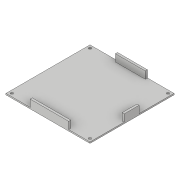
# Autodesk Inventor part: Board
Saved by Autodesk Inventor 2017 (Build 210142000, 142)
## iProperties
Created: 2019-06-10
Part Number: Board
Material: Generic
Document SubType Name: Modeling
Designer: markg
Density: 1 g/cm^3
Appearance: Default
Author: markg
Autodesk Inventor part; units mm, degrees
ref_plane "YZ Plane" through (0, 0, 0) normal (1, 0, 0) x (0, 1, 0)
ref_plane "XZ Plane" through (0, 0, 0) normal (0, 1, 0) x (-1, 0, 0)
ref_plane "XY Plane" through (0, 0, 0) normal (0, 0, 1) x (1, 0, 0)
sketch "Sketch1" plane through (0, 0, 0) normal (0, 1, 0) x (-1, 0, 0)
  line L0 (-50, 50) -> (50, 50)
  line L1 (50, 50) -> (50, -50)
  line L2 (50, -50) -> (-50, -50)
  line L3 (-50, -50) -> (-50, 50)
  line L4 (-50, 50) -> (50, -50) construction
  line L5 (50, 50) -> (-50, -50) construction
  circle A0 centre (46.444, 46.444) radius 1.5875
  circle A1 centre (46.444, -46.444) radius 1.5875
  circle A2 centre (-46.444, -46.444) radius 1.5875
  circle A3 centre (-46.444, 46.444) radius 1.5875
  point P0 (0, 0)
  dimension "d0" = 100
  dimension "d1" = 100
  dimension "d2" = 3.175
  dimension "d3" = 3.175
  dimension "d4" = 3.175
  dimension "d5" = 3.175
  dimension "d6" = 3.556
  dimension "d7" = 3.556
  dimension "d8" = 3.556
  dimension "d9" = 3.556
  constraints: 12 end point, 4 centre point, 4 point on line, 2 midpoint, 2 parallel, 1 horizontal, 1 perpendicular
  measures "d0" distance of L0.end L1.end
  measures "d1" distance of L1.end L2.end
  measures "d2" diameter of A0
  measures "d3" diameter of A1
  measures "d4" diameter of A2
  measures "d5" diameter of A3
  measures "d6" distance from line of L1 A0.centre
  measures "d7" distance from line of L1 A1.centre
  measures "d8" distance from line of L3 A2.centre
  measures "d9" distance from line of L3 A3.centre
extrude "Extrusion1" add sketch "Sketch1" along normal blind 1.5875
sketch "Sketch2" plane through (0, 1.5875, 0) normal (0, 1, 0) x (1, 0, 0)
  line L0 (-21.12, -50) -> (24.6, -50)
  line L1 (24.6, -50) -> (24.6, -47.46)
  line L2 (24.6, -47.46) -> (-21.12, -47.46)
  line L3 (-21.12, -47.46) -> (-21.12, -50)
  line L4 (50, 50) -> (-50, 50) projected
  line L5 (-17.31, 50) -> (18.25, 50)
  line L6 (18.25, 50) -> (18.25, 47.46)
  line L7 (18.25, 47.46) -> (-17.31, 47.46)
  line L8 (-17.31, 47.46) -> (-17.31, 50)
  line L9 (50, 8.42) -> (47.46, 8.42)
  line L10 (47.46, 8.42) -> (47.46, -9.36)
  line L11 (47.46, -9.36) -> (50, -9.36)
  line L12 (50, -9.36) -> (50, 8.42)
  line L13 (50, -50) -> (50, 50) projected
  line L14 (-50, -50) -> (50, -50) projected
  point P0 (0, 0)
  dimension "d12" = 2.54
  dimension "d13" = 2.54
  dimension "d14" = 2.54
  dimension "d15" = 0
  dimension "d16" = 0
  dimension "d17" = 25.4
  dimension "d18" = 45.72
  dimension "d19" = 17.78
  dimension "d20" = 35.56
  dimension "d21" = 40.64
  dimension "d22" = 31.75
  constraints: 24 end point, 6 parallel, 3 horizontal, 3 perpendicular, 1 point on line
  measures "d12" distance of L0.end L1.end
  measures "d13" distance of L9.start L9.end
  measures "d14" distance of L5.end L6.end
  measures "d15" distance between parallel lines of L13 L12
  measures "d16" distance between parallel lines of L14 L0
  measures "d17" distance between parallel lines of L13 L1
  measures "d18" distance of L1.end L2.end
  measures "d19" distance of L9.end L10.end
  measures "d20" distance of L6.end L7.end
  measures "d21" distance between parallel lines of L14 L11
  measures "d22" distance between parallel lines of L13 L6
extrude "Extrusion2" add sketch "Sketch2" along normal blind 8.509
body "Solid1"
